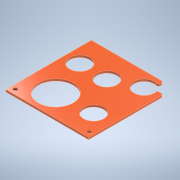
# Autodesk Inventor part: Bottle Spacer Base
Saved by Autodesk Inventor 2021 (Build 250183000, 183)
## iProperties
Created: 2020-08-14
Part Number: Bottle Spacer Base
Material: Generic
Document SubType Name: Modeling
Designer: jgray
Density: 1 g/cm^3
Appearance: Default
Author: jgray
Autodesk Inventor part; units mm, degrees
ref_plane "YZ Plane" through (0, 0, 0) normal (1, 0, 0) x (0, 1, 0)
ref_plane "XZ Plane" through (0, 0, 0) normal (0, 1, 0) x (-1, 0, 0)
ref_plane "XY Plane" through (0, 0, 0) normal (0, 0, 1) x (1, 0, 0)
sketch "Sketch1" plane through (0, 0, 0) normal (0, 1, 0) x (-1, 0, 0)
  circle A0 centre (18.5, 28) radius 23.85
  circle A1 centre (37, -23.25) radius 13.85
  arc A2 (-38.7137, -52.0928) -> (-48.6766, -40.9345) centre (-35, -38.75) ccw
  circle A3 centre (-30.9, 25.8) radius 13.85
  circle A4 centre (0, -23.25) radius 13.85
  line L0 (56.25, 58.25) -> (-56.25, 58.25)
  line L1 (-56.25, -58.25) -> (56.25, -58.25)
  line L2 (0, -105.9299) -> (0, 123.2086) construction
  line L3 (-76.4777, -38.75) -> (-5.35, -38.75) construction
  line L4 (-123.5447, -23.25) -> (82.5572, -23.25) construction
  line L5 (56.25, -58.25) -> (56.25, 58.25) construction
  line L6 (56.25, 58.25) -> (-56.25, 58.25)
  line L7 (-56.25, 58.25) -> (-56.25, -41.25)
  line L8 (-39.25, -58.25) -> (56.25, -58.25)
  line L9 (56.25, -58.25) -> (56.25, 58.25)
  line L10 (-56.25, -58.25) -> (-41.25, -58.25)
  line L11 (-41.25, -56.25) -> (-41.25, -54.0196)
  line L12 (-50.6516, -43.25) -> (-54.25, -43.25)
  line L13 (-56.25, -43.25) -> (-56.25, -58.25)
  arc A5 (-41.25, -56.25) -> (-39.25, -58.25) centre (-39.25, -56.25) ccw
  arc A6 (-56.25, -41.25) -> (-54.25, -43.25) centre (-54.25, -41.25) ccw
  arc A7 (-38.7137, -52.0928) -> (-41.25, -54.0196) centre (-39.25, -54.0196) ccw
  arc A8 (-50.6516, -43.25) -> (-48.6766, -40.9345) centre (-50.6516, -41.25) ccw
  point P0 (0, 0)
  point P1 (0, 0)
  point P2 (-48.0986, -43.25)
  point P3 (-56.25, -43.25)
  point P4 (-41.25, -51.1096)
  dimension "d0" = 47.7
  dimension "d1" = 27.7
  dimension "d2" = 27.7
  dimension "d3" = 27.7
  dimension "d4" = 27.7
  dimension "d5" = 116.5
  dimension "d6" = 112.5
  dimension "d7" = 37
  dimension "d8" = 18.5
  dimension "d9" = 30.9
  dimension "d10" = 19.5
  dimension "d11" = 35
  dimension "d12" = 35
  dimension "d13" = 25.8
  dimension "d14" = 28
  dimension "d20" = 112.5
  dimension "d21" = 56.25
  dimension "d22" = 58.25
  dimension "d23" = 116.5
  dimension "d24" = 23.25
  dimension "d25" = 35
  dimension "d26" = 35
  dimension "d27" = 19.25
  dimension "d28" = 37.75
  dimension "d29" = 30.25
  dimension "d30" = 2
  dimension "d31" = 2
  dimension "d32" = 15
  dimension "d33" = 15
  dimension "d34" = 2
  constraints: 28 end point, 12 point on circle, 11 point on line, 9 centre point, 8 tangent, 4 parallel, 3 horizontal, 3 perpendicular, 1 equal radius, 1 vertical
  measures "d0" diameter of A0
  measures "d1" diameter of A1
  measures "d2" diameter of A2
  measures "d3" diameter of A3
  measures "d4" diameter of A4
  measures "d5" distance between parallel lines of L0 L1
  measures "d6" distance of L1.start L1.end
  measures "d7" distance of A4.centre A1.centre
  measures "d8" distance from line of A0.centre L2
  measures "d9" distance from line of A3.centre L2
  measures "d10" distance between parallel lines of L1 L3
  measures "d11" distance between parallel lines of L1 L4
  measures "d12" horizontal distance of A2.centre A4.centre
  measures "d13" vertical distance of point (0, 0) A3.centre
  measures "d14" vertical distance of point (0, 0) A0.centre
  measures "d20" distance between parallel lines of L7 L5
  measures "d21" distance from line of point (0, 0) L5
  measures "d22" distance from line of L0 point (0, 0)
  measures "d23" distance between parallel lines of L1 L6
  measures "d24" distance from line of point (0, 0) L4
  measures "d25" distance from line of L1 A1.centre
  measures "d26" distance from line of L1 A4.centre
  measures "d27" distance from line of L9 A1.centre
  measures "d28" distance from line of A0.centre L5
  measures "d29" distance from line of L0 A0.centre
  measures "d30" radius of A5
  measures "d31" radius of A6
  measures "d32" distance between parallel lines of L13 L11
  measures "d33" distance between parallel lines of L1 L12
  measures "d34" radius of A7
extrude "Extrusion1" add sketch "Sketch1" along normal blind 3
sketch "Sketch2" plane through (0, 0, 0) normal (0, -1, 0) x (1, 0, 0)
  line L0 (70.8974, 51.25) -> (-70.9169, 51.25) construction
  line L1 (-56.25, 58.25) -> (56.25, 58.25) construction
  line L2 (56.25, 58.25) -> (56.25, -41.25) construction
  line L3 (-56.25, -58.25) -> (-56.25, 58.25) construction
  point P0 (0, 0)
  point P1 (50.25, 51.25)
  point P2 (-50.25, 51.25)
  dimension "d35" = 7
  dimension "d36" = 6
  dimension "d37" = 6
  constraints: 2 end point, 2 point on line, 1 horizontal
  measures "d35" distance between parallel lines of L0 L1
  measures "d36" distance from line of L2 point (50.25, 51.25)
  measures "d37" distance from line of L3 point (-50.25, 51.25)
hole "Hole1" at (50.25, 0, 51.25) at (-50.25, 0, 51.25) direction (0, 1, 0) diameter 5 end through all
sketch "Sketch3" plane through (-56.25, 0, 58.25) normal (0, 0, 1) x (1, 0, 0)
  line L0 (112.5, 0) -> (112.5, 3) projected
  line L1 (0, 0) -> (112.5, 0)
  line L2 (112.5, 0) -> (112.5, 3)
  line L3 (112.5, 3) -> (0, 3)
  line L4 (0, 3) -> (0, 0)
  point P0 (56.25, 0)
  constraints: 8 end point, 2 parallel, 1 horizontal, 1 perpendicular
extrude "Extrusion2" cut sketch "Sketch3" against normal blind 0.3
body "Solid1"
